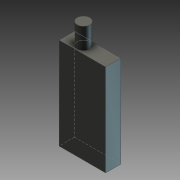
# Autodesk Inventor part: Video Tx
Saved by Autodesk Inventor 2012 (Build 160160000, 160)
## iProperties
Created: 2013-03-10
Part Number: Video Tx
Material: Default
Document SubType Name: Modeling
Designer: fixer
Density: 1.93984 g/cm^3
Mass: 21.5 g
Surface Area: 40.5514 cm^2
Volume: 11.0834 cm^3
Author: fixer
Autodesk Inventor part; units mm, degrees
ref_plane "YZ Plane" through (0, 0, 0) normal (1, 0, 0) x (0, 1, 0)
ref_plane "XZ Plane" through (0, 0, 0) normal (0, 1, 0) x (-1, 0, 0)
ref_plane "XY Plane" through (0, 0, 0) normal (0, 0, 1) x (1, 0, 0)
sketch "Sketch1" plane through (0, 0, 0) normal (0, 0, 1) x (1, 0, 0)
  line L0 (12.7, 25.019) -> (-12.7, 25.019)
  line L1 (-12.7, 25.019) -> (-12.7, -25.019)
  line L2 (-12.7, -25.019) -> (12.7, -25.019)
  line L3 (12.7, -25.019) -> (12.7, 25.019)
  point P0 (0, 0)
  point P1 (-12.7, 0)
  point P2 (0, 25.019)
  dimension "d0" = 25.4
  dimension "d1" = 50.038
  constraints: 8 end point, 2 midpoint, 2 parallel, 1 horizontal, 1 horizontal alignment, 1 perpendicular, 1 vertical alignment
  measures "d0" distance of L0.start L0.end
  measures "d1" distance of L0.end L1.end
extrude "Extrusion1" add sketch "Sketch1" along normal blind 8.382
sketch "Sketch2" plane through (-12.7, 25.019, 0) normal (0, 1, 0) x (1, 0, 0)
  line L0 (0, 0) -> (0, -8.382) projected
  circle A0 centre (9.144, -4.191) radius 3.4611
  point P0 (12.7, 0)
  dimension "d4" = 9.144
  constraints: 1 centre point
  measures "d4" distance from line of A0.centre L0
extrude "Extrusion2" add sketch "Sketch2" along normal blind 11.43
body "Solid1"
